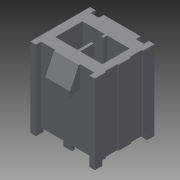
# Autodesk Inventor part: IPL1-102-01-S-K_header
Saved by Autodesk Inventor 2014 SP2 (Build 180246200, 246)
## iProperties
Created: 2019-03-13
Part Number: IPL1-102-01-S-K_header
Material: Generic
Catalog Web Link: www.cadenas.de
Description: IPL1--Header
Vendor: SAMTEC
Document SubType Name: Modeling
Designer: psadmin
Manufacturer: SAMTEC
Mass: 0.205945 g
Surface Area: 4.18515 cm^2
Volume: 0.205945 cm^3
Density: 1 g/cm^3
Appearance: PSOLRGB-175-175-175
Category: PARTsolutions
Company: SAMTEC
Title: IPL1-102-01-S-K_header
Author: Cadenas PARTsolutions
Comments: Header
PSOL_IDENT_0: {$CADENAS_DATA\23d-libs\samtec\modelling\ipl1\parts\ipl1_header.prj},210 {VTYP=3D},{NB=IPL1-102-01-S
PSOL_IDENT_1: -K_header},{LINA=IPL1-102-01-S-K_header},{NN=IPL1-},{DATE=31.07.2018 08:10:50},{GEOMDATE=31.07.2018
PSOL_IDENT_2: 07:23:50},{VERSION=},{LINEID=10},{WBVAR=POS,LS,ROPT,TOPT,POPT,WTOPT},{WBNUMERIC=}  {NB=IPL1-102-01-S
PSOL_IDENT_3: -K_header},{LINA=IPL1-102-01-S-K_header},{KT=DUMMY},{PN=IPL1-102-01-S-K},{SERIES=IPL1},{POSALG= '02'
PSOL_IDENT_4: , '-02' ,  '03' , '-03' , '04' , '-04' , '05' , '-05' , '06' , '-06' , '07' , '-07' , '08' , '-08'
PSOL_IDENT_5: ,  '09' , '-09' ,  '10' , '-10' ,  '11' , '-11' , '12' , '-12'  ,  '13' , '-13' ,  '14' , '-14' , '
PSOL_IDENT_6: 15' , '-15' , '16' , '-16'  ,  '17' , '-17' ,  '18' , '-18' , '19' , '-19' ,  '20' , '-20' ,  '21' ,
PSOL_IDENT_7: '-21' , '22' , '-22' , '23' , '-23' , '24' , '-24' ,  '25' , '-25'  },{POS=02},{LS=01},{ROPTALG=   '
PSOL_IDENT_8: S'  ,  '-S - Single Row'  ,   'D'  ,   '-D - Double Row'    },{ROPT=S},{TOPTALG=  ''  , 'Not Selecte
PSOL_IDENT_9: d'  ,   'RA'  , '-RA - Right Angle'   ,   'RE1'  , '-RE1 - Right Angle Elevated'   },{TOPT=},{POPTAL
PSOL_IDENT_10: G=  ''  ,  'Not Selected'  ,  'K'  ,  '-K - Keyed Polarization'  },{POPT=K},{WTOPTALG= '' , 'Not Ava
PSOL_IDENT_11: ilable' },{WTOPT=},{L=0.26000},{B=0.320},{E=0.230},{W=0.240},{PINS=2},{PINW=0.025},{PITCH=0.1000},{T
PSOL_IDENT_12: OPTPN=},{POPTPN=-K},{WTPN=},{PL=0.0000}
NN: IPL1-
NT: Header
NB: IPL1-102-01-S-K_header
NBSYN: $PN._header
LINA: IPL1-102-01-S-K_header
PN: IPL1-102-01-S-K
SERIES: IPL1
POS: -02
LS: -01
ROPT: -S - Single Row
TOPT: Not Selected
POPT: -K - Keyed Polarization
WTOPT: Not Available
L: 0.26
B: 0.32
E: 0.23
W: 0.24
PINS: 2
PINW: 0.025
PITCH: 0.1
SUPPLIER: SAMTEC
ARTICLENO: IPL1-102-01-S-K_header
BOMINFO: IPL1-102-01-S-K_header
CREATOR: CADENAS GmbH
Autodesk Inventor part; units mm, degrees
ref_plane "YZ Plane" through (0, 0, 0) normal (1, 0, 0) x (0, 1, 0)
ref_plane "XZ Plane" through (0, 0, 0) normal (0, 1, 0) x (-1, 0, 0)
ref_plane "XY Plane" through (0, 0, 0) normal (0, 0, 1) x (1, 0, 0)
sketch "Sketch_1" plane through (0, 0, 0) normal (1, 0, 0) x (0, 1, 0)
  line L0 (8.128, 3.048) -> (0, 3.048)
  line L1 (0, 3.048) -> (0, 2.286)
  line L2 (0, 2.286) -> (0.508, 2.286)
  line L3 (0.508, 2.286) -> (0.508, -2.286)
  line L4 (0.508, -2.286) -> (0, -2.286)
  line L5 (0, -2.286) -> (0, -3.048)
  line L6 (0, -3.048) -> (8.128, -3.048)
  line L7 (8.128, -3.048) -> (8.128, 3.048)
  constraints: 16 end point
extrude "Extrusion1" add sketch "Sketch_1" along normal mid plane 6.604
sketch "Sketch_4" plane through (0, 0, 0) normal (0, 0, 1) x (1, 0, 0)
  line L0 (-2.7305, 0.508) -> (-2.7305, -0.508)
  line L1 (-2.7305, -0.508) -> (-0.4445, -0.508)
  line L2 (-0.4445, -0.508) -> (-0.4445, 0.508)
  line L3 (-0.4445, 0.508) -> (-2.7305, 0.508)
  constraints: 8 end point
extrude "Extrusion2" cut sketch "Sketch_4" along normal mid plane 6.096
sketch "Sketch_5" plane through (0, 0, 0) normal (0, 0, 1) x (1, 0, 0)
  line L0 (0.4445, 0.508) -> (0.4445, -0.508)
  line L1 (0.4445, -0.508) -> (2.7305, -0.508)
  line L2 (2.7305, -0.508) -> (2.7305, 0.508)
  line L3 (2.7305, 0.508) -> (0.4445, 0.508)
  constraints: 8 end point
extrude "Extrusion3" cut sketch "Sketch_5" along normal mid plane 6.096
sketch "Sketch_9" plane through (0, 8.128, 0) normal (0, 1, 0) x (1, 0, 0)
  line L0 (-2.4117, 1.3945) -> (-2.4117, -1.397)
  line L1 (-2.4117, -1.397) -> (-0.1283, -1.397)
  line L2 (-0.1283, -1.397) -> (-0.1283, 1.3945)
  line L3 (-0.1283, 1.3945) -> (-2.4117, 1.3945)
  constraints: 8 end point
extrude "Extrusion4" cut sketch "Sketch_9" against normal blind 5.842
pattern_linear "Rectangular Pattern1" count 2 spacing 2.54 along (0.9999995, 0, -0.001) of "Extrusion4"
sketch "Sketch_21" plane through (0, 0, 0) normal (0, 1, 0) x (-1, 0, 0)
  line L0 (3.81, -3.81) -> (3.81, 3.556)
  line L1 (3.81, 3.556) -> (-3.81, 3.556)
  line L2 (-3.81, 3.556) -> (-3.81, -3.81)
  line L3 (-3.81, -3.81) -> (3.81, -3.81)
  line L4 (3.302, -3.048) -> (3.302, 3.048)
  line L5 (3.302, 3.048) -> (2.7305, 3.048)
  line L6 (2.7305, 3.048) -> (2.7305, 2.54)
  line L7 (2.7305, 2.54) -> (-2.7305, 2.54)
  line L8 (-2.7305, 2.54) -> (-2.7305, 3.048)
  line L9 (-2.7305, 3.048) -> (-3.302, 3.048)
  line L10 (-3.302, 3.048) -> (-3.302, -3.048)
  line L11 (-3.302, -3.048) -> (-2.7305, -3.048)
  line L12 (-2.7305, -3.048) -> (-2.7305, -2.54)
  line L13 (-2.7305, -2.54) -> (-1.905, -2.54)
  line L14 (-1.905, -2.54) -> (-1.905, -3.048)
  line L15 (-1.905, -3.048) -> (1.905, -3.048)
  line L16 (1.905, -3.048) -> (1.905, -2.54)
  line L17 (1.905, -2.54) -> (2.7305, -2.54)
  line L18 (2.7305, -2.54) -> (2.7305, -3.048)
  line L19 (2.7305, -3.048) -> (3.302, -3.048)
  constraints: 40 end point
extrude "Extrusion5" cut sketch "Sketch_21" along normal blind 8.128
sketch "Sketch_25" plane through (0, 0, 0) normal (1, 0, 0) x (0, 1, 0)
  line L0 (6.223, 3.556) -> (5.6388, 3.556)
  line L1 (5.6388, 3.556) -> (5.9182, 2.794)
  line L2 (5.9182, 2.794) -> (5.9182, 2.54)
  line L3 (5.9182, 2.54) -> (8.128, 2.54)
  line L4 (8.128, 2.54) -> (8.128, 2.667)
  line L5 (8.128, 2.667) -> (6.223, 3.556)
  constraints: 12 end point
extrude "Extrusion6" add sketch "Sketch_25" along normal mid plane 2.54
sketch "Sketch_26" plane through (0, 8.128, 0) normal (0, 1, 0) x (1, 0, 0)
  line L0 (-0.508, 1.016) -> (-0.508, 0)
  line L1 (-0.508, 0) -> (0.508, 0)
  line L2 (0.508, 0) -> (0.508, 1.016)
  line L3 (0.508, 1.016) -> (-0.508, 1.016)
  constraints: 8 end point
extrude "Extrusion7" cut sketch "Sketch_26" against normal blind 5.842
sketch "Sketch_38" plane through (0, 0, 0) normal (0, 1, 0) x (-1, 0, 0)
  line L0 (-3.175, 0.635) -> (-3.175, 1.905)
  line L1 (-3.175, 1.905) -> (-3.556, 1.905)
  line L2 (-3.556, 1.905) -> (-3.556, -1.905)
  line L3 (-3.556, -1.905) -> (-3.175, -1.905)
  line L4 (-3.175, -1.905) -> (-3.175, -0.635)
  line L5 (-3.175, -0.635) -> (-3.429, -0.635)
  line L6 (-3.429, -0.635) -> (-3.429, 0.635)
  line L7 (-3.429, 0.635) -> (-3.175, 0.635)
  constraints: 16 end point
extrude "Extrusion8" cut sketch "Sketch_38" along normal blind 8.128
ref_plane "header_to_dummy_XY" through (0, 0, 0) normal (0, -1, 0) x (1, 0, 0)
ref_plane "header_to_dummy_YZ" through (0, 0, 0) normal (1, 0, 0) x (0, 0, 1)
ref_plane "header_to_dummy_ZX" through (0, 0, 0) normal (0, 0, 1) x (0, -1, 0)
ref_plane "header_to_pad_XY" through (0, 8.128, 0) normal (0, 1, 0) x (1, 0, 0)
ref_plane "header_to_pad_YZ" through (0, 8.128, 0) normal (1, 0, 0) x (0, 0, -1)
ref_plane "header_to_pad_ZX" through (0, 8.128, 0) normal (0, 0, -1) x (0, 1, 0)
body "Solid1"
